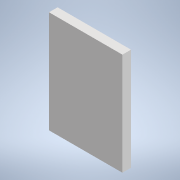
# Autodesk Inventor part: topOfLiftFrame
Saved by Autodesk Inventor 2020.2 (Build 242310000, 310)
## iProperties
Created: 2020-01-07
Part Number: topOfLiftFrame
Material: Generic
Document SubType Name: Modeling
Designer: steele
Density: 1 g/cm^3
Appearance: Default
Author: steele
Autodesk Inventor part; units mm, degrees
ref_plane "YZ Plane" through (0, 0, 0) normal (1, 0, 0) x (0, 1, 0)
ref_plane "XZ Plane" through (0, 0, 0) normal (0, 1, 0) x (-1, 0, 0)
ref_plane "XY Plane" through (0, 0, 0) normal (0, 0, 1) x (1, 0, 0)
sketch "Sketch1" plane through (0, 0, 0) normal (0, 0, 1) x (1, 0, 0)
  line L0 (-53.975, 0) -> (-53.975, -6.35) projected
  line L1 (0, -6.35) -> (-53.975, -6.35) projected
  line L2 (0, 0) -> (0, -6.35) projected
  line L3 (-53.975, 0) -> (0, 0) projected
  line L4 (-53.975, 68.834) -> (-53.975, 62.484) projected
  line L5 (0, 62.484) -> (-53.975, 62.484) projected
  line L6 (0, 68.834) -> (0, 62.484) projected
  line L7 (-53.975, 68.834) -> (0, 68.834) projected
  line L8 (-53.975, 68.834) -> (0, 68.834)
  line L9 (0, 68.834) -> (0, -6.35)
  line L10 (0, -6.35) -> (-53.975, -6.35)
  line L11 (-53.975, -6.35) -> (-53.975, 68.834)
  constraints: 8 end point, 2 parallel, 1 horizontal, 1 perpendicular
extrude "Extrusion1" add sketch "Sketch1" along normal blind 6.35
body "Solid1"
